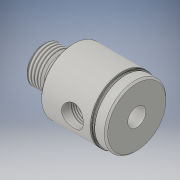
# Autodesk Inventor part: 09R000-0_rod_guide
Saved by Autodesk Inventor 2016 SP1 (Build 200210100, 210)
## iProperties
Category: PARTsolutions
Company: BIMBA
Created: 2017-03-15
Part Number: 09R000-0_rod_guide
Material: Generic
Catalog Web Link: www.cadenas.de
Description: Rod Guide-Original Line - Standard Air Cylinders
Vendor: BIMBA
Document SubType Name: Standard Catalog Part
Designer: 589013
Manufacturer: BIMBA
Mass: 17.0993 g
Surface Area: 57.1191 cm^2
Volume: 17.0993 cm^3
Density: 1 g/cm^3
Appearance: PSOLRGB-211-211-211
PSOL_IDENT_0: {$CADENAS_DATA\23d-libs\bimba\bimba\bimba_imperial\bimba_full_line\original_line_cylinders\standard_
PSOL_IDENT_1: air_cylinders\rod_guide.prj},232 {VTYP=3D},{NB=09R000-0_rod_guide},{LINA=09R000-0_rod_guide},{NN=Rod
PSOL_IDENT_2: Guide},{DATE=09.11.2016 07:55:11},{GEOMDATE=07.11.2015 13:30:00},{VERSION=},{LINEID=60},{LINESUBID=
PSOL_IDENT_3: -1},{WBVAR=MNT,ACTING,NR,K,Q,T1,T2,T3,T4,MB,TRIM,CUSH,RODTRANS}  {NB=09R000-0_rod_guide},{LINA=09R00
PSOL_IDENT_4: 0-0_rod_guide},{KT=DUMMY},{PN=09R000},{BORE=1.06250000},{BOREPN=09},{MNT=},{MNTALG='' , 'Front Nose'
PSOL_IDENT_5: , 'BF' , 'Front Block' , 'BFT' , 'Front Trunnion' , 'A' , 'Adjustable Stroke'},{ACTING=R},{ACTINGAL
PSOL_IDENT_6: G= '' , 'Single Acting' , 'R' , 'Reverse/Double Acting' },{NR=},{NRALG= '' , 'N/A' },{K=},{Q=},{QALG=
PSOL_IDENT_7: '' , 'Without Side Ported Rear Head' , 'Q' , 'With Side Ported Rear Head' },{T1=},{T2=},{T3=},{T4=}
PSOL_IDENT_8: ,{MB=0},{A1=1.6250},{A1N=1.0000},{A1P=1.6250},{A1B=1.8750},{A2=0.5000},{A2N=0.5000},{A2P=0.5000},{A3=
PSOL_IDENT_9: 0.8750},{A3N=0.1250},{A3P=0.8750},{A4=0.2525},{A4N=0.3750},{A4P=0.2525},{A5=0.0300},{A6=0.0000},{A6N=
PSOL_IDENT_10: 0.1250},{A6P=0.0000},{A7=0.2550},{A7N=0.3320},{A7P=0.2550},{A8=0.0300},{A8N=0.0300},{A8NR=0.0300},{D
PSOL_IDENT_11: 1=1.1130},{D1N=1.1130},{D1P=1.1130},{D1B=1.1410},{D2=1.0715},{D3=0.0000},{D3N=0.8120},{D3P=0.0000},{
PSOL_IDENT_12: D4=0.7500},{D4N=0.3390},{D4P=0.7500},{D4NR=0.3775},{D5=0.3160},{D5N=0.3160},{D5NR=0.3775},{C1=0.030}
PSOL_IDENT_13: ,{C2=0.0300},{C2N=0.0300},{C2P=0.0300},{C3=0.0000},{C3N=0.0000},{C3P=0.0000},{C4=0.0300},{C4N=0.0300
PSOL_IDENT_14: },{C4P=0.0300},{NDM=0.6250},{NDMN=0.6250},{NDMP=0.6250},{TAB=UNF},{D6=0.6225},{D6N=0.6225},{D6P=0.62
PSOL_IDENT_15: 25},{A9=0.0940},{A9N=0.0940},{A9P=0.0940},{D7=0.5385},{D7N=0.5385},{D7P=0.5385},{A10=0.0855},{A10N=0
PSOL_IDENT_16: .0855},{A10P=0.0855},{R1=0.0350},{R1N=0.0350},{R1P=0.0350},{D8=0.6560},{D9=0.6250},{D10=0.5620},{A11=
PSOL_IDENT_17: 0.7710},{A12=0.8340},{A13=0.9900},{A14=0.5620},{A14N=0.5620},{A14B=0.6250},{D11=0.2500},{D11N=0.2500
PSOL_IDENT_18: },{NDM2=0.4050},{NDM2N=0.4050},{NDM2DP=0.3750},{THREAD=0},{HEX=0.3775},{HEXN=0.3775},{S1=1.2500},{B1=
PSOL_IDENT_19: 0.1275},{B2=0.7190},{B22=0.0000},{DB=0.0000},{B3=0.3120},{B4=0.8127},{X1=0.0920},{X2=0.7475},{NDM3=0
PSOL_IDENT_20: .2500},{NDM4=0.1900},{NDM4DP=0.3100},{DD=1.2500},{CB=0.3280},{CBDP=0.2190},{PORT=1},{XT=0.7170},{XTX=
PSOL_IDENT_21: 0.7170},{XT1=0.5000},{XT2=0.3800},{NDMH=0.6250},{OD=1.1130},{ID=1.0715},{G=0.0000},{PNUT=0.4060},{TR
PSOL_IDENT_22: IM=0},{C11=0.2775},{C22=0.4045},{C33=0.2450},{C44=0.5350},{C55=0.7000},{CD1=0.2050},{CD2=0.1360},{CD
PSOL_IDENT_23: 3=0.0775},{CNDM3=0.1900},{CTAB3=UNS},{CUSH=0},{XX=0.81270},{LCD=0.0000},{RODTRANS=0.00000}
NN: Rod Guide
NT: Original Line - Standard Air Cylinders
NB: 09R000-0_rod_guide
NBSYN: $PN.-$RODTRANS._rod_guide
LINA: 09R000-0_rod_guide
BORE: 1 1/16
BOREPN: 09
MNT: Front Nose
MNTALG: '' , 'Front Nose' , 'BF' , 'Front Block' , 'BFT' , 'Front Trunnion' , 'A' , 'Adjustable Stroke'
ACTING: Reverse/Double Acting
NR: N/A
K: Standard
Q: Without Side Ported Rear Head
T1: without T1
T2: without T2
T3: without T3
T4: without T4
MB: 0
A1N: 1.0000
A1P: 1.6250
A1B: 1.8750
A2N: 0.5000
A2P: 0.5000
A3N: 0.1250
A3P: 0.8750
A4N: 0.3750
A4P: 0.2525
A5: 0.0300
A6N: 0.1250
A6P: 0.0000
A7N: 0.3320
A7P: 0.2550
A8N: 0.0300
A8NR: 0.0300
D1N: 1.1130
D1P: 1.1130
D1B: 1.1410
D2: 1.0715
D3N: 0.8120
D3P: 0.0000
D4N: 0.3390
D4P: 0.7500
D4NR: 0.3775
D5N: 0.3160
D5NR: 0.3775
C1: 0.030
C2N: 0.0300
C2P: 0.0300
C3N: 0.0000
C3P: 0.0000
C4N: 0.0300
C4P: 0.0300
NDMN: 0.6250
NDMP: 0.6250
TAB: UNF
D6N: 0.6225
D6P: 0.6225
A9N: 0.0940
A9P: 0.0940
D7N: 0.5385
D7P: 0.5385
A10N: 0.0855
A10P: 0.0855
R1N: 0.0350
R1P: 0.0350
D8: 0.6560
D9: 0.6250
D10: 0.5620
A11: 0.7710
A12: 0.8340
A13: 0.9900
A14N: 0.5620
A14B: 0.6250
D11N: 0.2500
NDM2N: 0.4050
NDM2DP: 0.3750
HEXN: 0.3775
S1: 1.2500
B1: 0.1275
B2: 0.7190
B22: 0.0000
DB: 0.0000
B3: 0.3120
B4: 0.8127
X1: 0.0920
X2: 0.7475
NDM3: 0.2500
NDM4: 0.1900
NDM4DP: 0.3100
DD: 1.2500
CB: 0.3280
CBDP: 0.2190
XTX: 0.7170
XT1: 0.5000
XT2: 0.3800
NDMH: 0.6250
TRIM: 0
C11: 0.2775
C22: 0.4045
C33: 0.2450
C44: 0.5350
C55: 0.7000
CD1: 0.2050
CD2: 0.1360
CD3: 0.0775
CNDM3: 0.1900
CTAB3: UNS
CUSH: 0
LCD: 0.0000
RODTRANS: 0.00000
SUPPLIER: BIMBA
ARTICLENO: 09R000-0_rod_guide
BOMINFO: 09R000-0_rod_guide
CREATOR: CADENAS GmbH
Title: 09R000-0_rod_guide
Author: Cadenas PARTsolutions
Comments: Original Line - Standard Air Cylinders
Autodesk Inventor part; units mm, degrees
sketch "Sketch_2" plane through (0, 0, 0) normal (0, 0, 1) x (1, 0, 0)
  line L0 (12.7, 0) -> (0, 0)
  line L1 (0, 0) -> (0, 7.098)
  line L2 (0, 7.098) -> (0.8395, 7.9375)
  line L3 (0.8395, 7.9375) -> (6.6726, 7.9375)
  line L4 (6.6726, 7.9375) -> (7.5126, 7.0988)
  arc A0 (7.5126, 7.0988) -> (8.1407, 6.839) centre (8.1407, 7.728) ccw
  line L5 (8.1407, 6.839) -> (9.4234, 6.839)
  arc A1 (9.4234, 6.839) -> (10.3124, 7.7279) centre (9.4234, 7.7279) ccw
  line L6 (10.3124, 7.7279) -> (10.3124, 7.9057)
  line L7 (10.3124, 7.9057) -> (12.7, 7.9057)
  line L8 (12.7, 7.9057) -> (12.7, 0)
  line L9 (12.7, 0) -> (0, 0)
  constraints: 20 end point, 4 point on circle, 2 centre point
revolve "Revolution1" add sketch "Sketch_2" angle 360 about axis through (12.7, 0, 0) along (1, 0, 0)
thread "Thread1" size "5/8-18 UNF" class "2A" standard "ANSI Unified Screw Threads" full length
sketch "Sketch_3" plane through (0, 0, 0) normal (0, 0, 1) x (1, 0, 0)
  line L0 (41.275, 0) -> (12.7, 0)
  line L1 (12.7, 0) -> (12.7, 13.3731)
  line L2 (12.7, 13.3731) -> (13.462, 14.1351)
  line L3 (13.462, 14.1351) -> (34.8615, 14.1351)
  line L4 (34.8615, 14.1351) -> (34.8615, 12.846)
  line L5 (34.8615, 12.846) -> (35.6235, 12.846)
  line L6 (35.6235, 12.846) -> (36.3855, 13.6081)
  line L7 (36.3855, 13.6081) -> (40.513, 13.6081)
  line L8 (40.513, 13.6081) -> (41.275, 12.846)
  line L9 (41.275, 12.846) -> (41.275, 0)
  line L10 (41.275, 0) -> (12.7, 0)
  constraints: 22 end point
revolve "Revolution2" add sketch "Sketch_3" angle 360 about axis through (41.275, 0, 0) along (1, 0, 0)
sketch "Sketch3" plane through (0, 0, 0) normal (-1, 0, 0) x (0, 0, 1)
  point P0 (0, 0)
hole "Hole1" at (0, 0, 0) direction (1, 0, 0) diameter 8.0264 depth 41.275 countersink diameter 9.5504 countersink angle 90
sketch "Sketch_40" plane through (0, 0, 0) normal (0, 1, 0) x (-1, 0, 0)
  line L0 (-27.0002, 14.1351) -> (-27.0002, 0)
  line L1 (-27.0002, 0) -> (-30.1752, 0)
  line L2 (-30.1752, 0) -> (-30.1752, 3.243)
  line L3 (-30.1752, 3.243) -> (-31.5423, 4.6101)
  line L4 (-31.5423, 4.6101) -> (-31.8397, 14.1351)
  line L5 (-31.8397, 14.1351) -> (-27.0002, 14.1351)
  line L6 (-27.0002, 14.1351) -> (-27.0002, 0)
  constraints: 14 end point
revolve "Revolution3" cut sketch "Sketch_40" angle 360 about axis through (27.0002, 0, 14.1351) along (0, 0, 1)
thread "Thread2" size "1/8" designation "1/8 - 27 NPT" standard "NPT" length 5.7178
sketch "Sketch_47" plane through (0, 0, 0) normal (0, 0, 1) x (1, 0, 0)
  line L0 (35.6235, 0) -> (34.8615, 0)
  line L1 (34.8615, 13.449) -> (34.8615, 12.5921)
  line L2 (34.8615, 12.5921) -> (35.6235, 12.5921)
  line L3 (35.6235, 12.5921) -> (35.6235, 12.846)
  line L4 (35.6235, 12.846) -> (35.2425, 12.846)
  line L5 (35.2425, 12.846) -> (34.984, 13.1046)
  arc A0 (34.984, 13.2842) -> (34.984, 13.1046) centre (35.0738, 13.1944) ccw
  line L6 (34.984, 13.2842) -> (35.7508, 14.0509)
  line L7 (35.7508, 14.0509) -> (35.7508, 14.1351)
  line L8 (35.7508, 14.1351) -> (35.5476, 14.1351)
  line L9 (35.5476, 14.1351) -> (34.8615, 13.449)
  constraints: 20 end point, 2 point on circle, 1 centre point
revolve "Revolution4" add sketch "Sketch_47" angle 360 about axis through (35.6235, 0, 0) along (1, 0, 0)
ref_plane "dp1_XY" through (12.7, 7.9057, 0) normal (0, 0, 1) x (1, 0, 0)
ref_plane "dp1_YZ" through (12.7, 7.9057, 0) normal (1, 0, 0) x (0, 1, 0)
ref_plane "dp1_ZX" through (12.7, 7.9057, 0) normal (0, 1, 0) x (0, 0, 1)
ref_plane "dp2_XY" through (12.7, -7.9057, 0) normal (0, 0, 1) x (1, 0, 0)
ref_plane "dp2_YZ" through (12.7, -7.9057, 0) normal (1, 0, 0) x (0, 1, 0)
ref_plane "dp2_ZX" through (12.7, -7.9057, 0) normal (0, 1, 0) x (0, 0, 1)
ref_plane "hh_XY" through (0, 7.9375, 0) normal (0, 0, 1) x (1, 0, 0)
ref_plane "hh_YZ" through (0, 7.9375, 0) normal (1, 0, 0) x (0, 1, 0)
ref_plane "hh_ZX" through (0, 7.9375, 0) normal (0, 1, 0) x (0, 0, 1)
ref_plane "port_XY" through (27.0002, 0, 0) normal (0, 0, 1) x (1, 0, 0)
ref_plane "port_YZ" through (27.0002, 0, 0) normal (1, 0, 0) x (0, 1, 0)
ref_plane "port_ZX" through (27.0002, 0, 0) normal (0, 1, 0) x (0, 0, 1)
ref_plane "rod_guide_XY" through (0, 0, 0) normal (1, 0, 0) x (0, 0, -1)
ref_plane "rod_guide_YZ" through (0, 0, 0) normal (0, 0, -1) x (0, 1, 0)
ref_plane "rod_guide_ZX" through (0, 0, 0) normal (0, 1, 0) x (1, 0, 0)
ref_plane "s1_XY" through (10.3124, 0, 0) normal (0, 0, 1) x (1, 0, 0)
ref_plane "s1_YZ" through (10.3124, 0, 0) normal (1, 0, 0) x (0, 1, 0)
ref_plane "s1_ZX" through (10.3124, 0, 0) normal (0, 1, 0) x (0, 0, 1)
ref_plane "s2_XY" through (12.7, 0, 0) normal (0, 0, 1) x (1, 0, 0)
ref_plane "s2_YZ" through (12.7, 0, 0) normal (1, 0, 0) x (0, 1, 0)
ref_plane "s2_ZX" through (12.7, 0, 0) normal (0, 1, 0) x (0, 0, 1)
ref_plane "t1_XY" through (12.7, 0, 0) normal (1, 0, 0) x (0, 0, -1)
ref_plane "t1_YZ" through (12.7, 0, 0) normal (0, 0, -1) x (0, 1, 0)
ref_plane "t1_ZX" through (12.7, 0, 0) normal (0, 1, 0) x (1, 0, 0)
ref_plane "t111_XY" through (12.7, 0, 0) normal (1, 0, 0) x (0, 0, -1)
ref_plane "t111_YZ" through (12.7, 0, 0) normal (0, 0, -1) x (0, 1, 0)
ref_plane "t111_ZX" through (12.7, 0, 0) normal (0, 1, 0) x (1, 0, 0)
ref_plane "to_foot_bracket_XY" through (12.7, 0, 0) normal (1, 0, 0) x (0, 0, -1)
ref_plane "to_foot_bracket_YZ" through (12.7, 0, 0) normal (0, 0, -1) x (0, 1, 0)
ref_plane "to_foot_bracket_ZX" through (12.7, 0, 0) normal (0, 1, 0) x (1, 0, 0)
ref_plane "to_nut_XY" through (10.3124, 0, 0) normal (1, 0, 0) x (0, 0, -1)
ref_plane "to_nut_YZ" through (10.3124, 0, 0) normal (0, 0, -1) x (0, 1, 0)
ref_plane "to_nut_ZX" through (10.3124, 0, 0) normal (0, 1, 0) x (1, 0, 0)
ref_plane "to_rod_XY" through (0, 0, 0) normal (1, 0, 0) x (0, 0, -1)
ref_plane "to_rod_YZ" through (0, 0, 0) normal (0, 0, -1) x (0, 1, 0)
ref_plane "to_rod_ZX" through (0, 0, 0) normal (0, 1, 0) x (1, 0, 0)
ref_plane "to_screw_XY" through (27.0002, 10.2743, -7.0485) normal (0, 1, 0) x (1, 0, 0)
ref_plane "to_screw_YZ" through (27.0002, 10.2743, -7.0485) normal (1, 0, 0) x (0, 0, -1)
ref_plane "to_screw_ZX" through (27.0002, 10.2743, -7.0485) normal (0, 0, -1) x (0, 1, 0)
ref_plane "to_trunnion_brackets_XY" through (18.2118, 0, 0) normal (0, 1, 0) x (1, 0, 0)
ref_plane "to_trunnion_brackets_YZ" through (18.2118, 0, 0) normal (1, 0, 0) x (0, 0, -1)
ref_plane "to_trunnion_brackets_ZX" through (18.2118, 0, 0) normal (0, 0, -1) x (0, 1, 0)
ref_plane "to_trunnion_brackets1_XY" through (18.2118, 15.875, 0) normal (0, 1, 0) x (1, 0, 0)
ref_plane "to_trunnion_brackets1_YZ" through (18.2118, 15.875, 0) normal (1, 0, 0) x (0, 0, -1)
ref_plane "to_trunnion_brackets1_ZX" through (18.2118, 15.875, 0) normal (0, 0, -1) x (0, 1, 0)
ref_plane "to_trunnion_brackets2_XY" through (18.2118, -15.875, 0) normal (0, 1, 0) x (1, 0, 0)
ref_plane "to_trunnion_brackets2_YZ" through (18.2118, -15.875, 0) normal (1, 0, 0) x (0, 0, -1)
ref_plane "to_trunnion_brackets2_ZX" through (18.2118, -15.875, 0) normal (0, 0, -1) x (0, 1, 0)
ref_plane "to_tube_XY" through (35.6235, 0, 0) normal (1, 0, 0) x (0, 0, -1)
ref_plane "to_tube_YZ" through (35.6235, 0, 0) normal (0, 0, -1) x (0, 1, 0)
ref_plane "to_tube_ZX" through (35.6235, 0, 0) normal (0, 1, 0) x (1, 0, 0)
body "Solid1"
